table_thing (Autodesk Fusion 360 design; units mm, degrees)
Autodesk Fusion 360 part; units mm, degrees
sketch "Sketch1" plane through (0, 0, 0) normal (0, 1, 0) x (1, 0, 0)
  line L0 (0, 0) -> (-80, 0)
  line L1 (-80, 0) -> (-80, -40)
  line L2 (-80, -40) -> (0, -40)
  line L3 (0, -40) -> (0, 0)
  dimension "d1" = 40
  dimension "d2" = 80
  constraint horizontal L0
  constraint vertical L1
  constraint horizontal L2
  constraint vertical L3
  constraint coincident L0.start L3.end
  measures "d1" distance of L0.start L2.end
  measures "d2" distance of L0.start L0.end
extrude "Extrude1" add sketch "Sketch1" along normal blind 30
fillet "Fillet1" radius 3 4 edges at (0, 15, 40) (-80, 15, 40) (0, 15, 0) (-80, 15, 0)
ref_plane "WorkPlane1" through (-40, 15, 20) normal (0, 0, 1) x (1, 0, 0)
sketch "Sketch2" plane through (0, 0, 20) normal (0, 0, 1) x (1, 0, 0)
  spline S0 degree 5 poles (0, 30) (-1.6, 29.3932) (-4.8, 28.2326) (-9.6, 26.6508) (-16, 24.8648) (-24, 23.2075) (-32, 22.1769) (-40, 21.824) (-48, 22.1769) (-56, 23.2075) (-64, 24.8648) (-70.4, 26.6508) (-75.2, 28.2326) (-78.4, 29.3932) (-80, 30) knots 0 0 0 0 0 0 0.1 0.2 0.3 0.4 0.5 0.6 0.7 0.8 0.9 1 1 1 1 1 1
  line L0 (0, 0) -> (0, 30)
  line L1 (-80, 30) -> (-80, 0)
  line L2 (0, 0) -> (-80, 0)
  line L3 (0, 30) -> (-80, 30)
  line L4 (-40, 22) -> (-40, 30)
  point P0 (-40, 22)
  dimension "d8" = 80
  dimension "d9" = 22
  constraint coincident L0.start L2.start
  constraint vertical L0
  constraint parallel L0 L1
  constraint perpendicular L1 L2
  constraint perpendicular L1 L3
  constraint coincident P0 L4.start
  constraint midpoint L3 L4.end
  constraint perpendicular L3 L4
  measures "d8" distance of L1.end L0.start
  measures "d9" distance of P0 L2
sketch "Sketch3" plane through (-80, 0, 0) normal (-1, 0, 0) x (0, -1, 0)
  line L0 (-30, 3) -> (0, 3)
  line L1 (0, 3) -> (0, 37)
  line L2 (0, 37) -> (-30, 37)
  line L3 (-30, 37) -> (-30, 3)
  line L4 (0, 0) -> (-41.6248, 0)
  line L5 (-41.6248, 0) -> (-41.6248, 40)
  line L6 (-41.6248, 40) -> (0, 40)
  line L7 (0, 40) -> (0, 0)
  spline S0 degree 5 poles (-41.6248, 40) (-40.7431, 39.704) (-39.0566, 39.0064) (-36.758, 37.6429) (-34.1628, 35.1825) (-31.7546, 31.0174) (-30.257, 25.8742) (-29.7443, 20) (-30.257, 14.1258) (-31.7546, 8.9826) (-34.1628, 4.8175) (-36.758, 2.3571) (-39.0566, 0.9936) (-40.7431, 0.296) (-41.6248, 0) knots 0 0 0 0 0 0 0.1 0.2 0.3 0.4 0.5 0.6 0.7 0.8 0.9 1 1 1 1 1 1
  line L8 (-30, 25) -> (-30, 15)
  point P0 (-30, 20)
  dimension "d10" = 40
  constraint coincident L4.start L7.end
  constraint horizontal L4
  constraint perpendicular L4 L5
  constraint perpendicular L5 L6
  constraint perpendicular L4 L7
  constraint midpoint L3 P0
  constraint midpoint P0 L8
  constraint coincident L3 L8.start
  measures "d10" distance of L6.end L4.start
sweep "Sweep1" cut profiles "Sketch3" path "Sketch2" along S0 section 1 contours L5 S0
